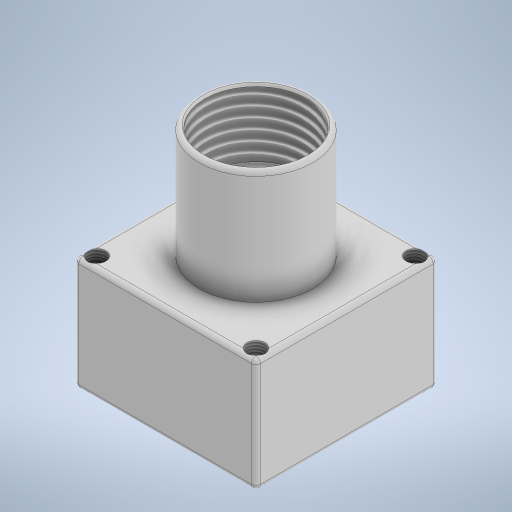
# Autodesk Inventor part: PRACTICA #1 CONOCIENDO INVENTOR CARLOS LUCERO NO. 1184321
Saved by Autodesk Inventor 2024 (Build 280153000, 153)
## iProperties
Created: 2024-01-26
Part Number: PRACTICA #1 CONOCIENDO INVENTOR CARLOS LUCERO NO. 1184321
Material: Genérico
Document SubType Name: Modeling
Designer: Andres
Density: 1 g/cm^3
Appearance: Valor por defecto
Author: Andres
Autodesk Inventor part; units mm, degrees
ref_plane "YZ Plane" through (0, 0, 0) normal (1, 0, 0) x (0, 1, 0)
ref_plane "XZ Plane" through (0, 0, 0) normal (0, 1, 0) x (-1, 0, 0)
ref_plane "XY Plane" through (0, 0, 0) normal (0, 0, 1) x (1, 0, 0)
sketch "Boceto1" plane through (0, 0, 0) normal (0, 1, 0) x (-1, 0, 0)
  line L0 (40, 40) -> (-40, 40)
  line L1 (-40, 40) -> (-40, -40)
  line L2 (-40, -40) -> (40, -40)
  line L3 (40, -40) -> (40, 40)
  line L4 (40, 40) -> (-40, -40) construction
  line L5 (-40, 40) -> (40, -40) construction
  point P0 (0, 0)
  dimension "d0" = 80
  dimension "d1" = 80
  constraints: 12 end point, 2 midpoint, 2 parallel, 1 horizontal, 1 perpendicular
  measures "d0" distance of L0.start L0.end
  measures "d1" distance of L1.end L0.end
extrude "Extrusión1" add sketch "Boceto1" along normal blind 50
sketch "Boceto2" plane through (0, 50, 0) normal (0, 1, 0) x (1, 0, 0)
  circle A0 centre (0, 0) radius 25
  circle A1 centre (0, 0) radius 22.5
  dimension "d4" = 50
  dimension "d5" = 45
  constraints: 2 centre point, 2 coincident
  measures "d4" diameter of A0
  measures "d5" diameter of A1
extrude "Extrusión2" add sketch "Boceto2" along normal blind 50 contours A0 | A1
sketch "Boceto3" plane through (0, 100, 0) normal (0, 1, 0) x (1, 0, 0)
  circle A0 centre (0, 0) radius 22.5
  dimension "d8" = 45
  constraints: 1 centre point, 1 coincident
  measures "d8" diameter of A0
extrude "Extrusión3" cut sketch "Boceto3" against normal blind 30
sketch "Boceto4" plane through (0, 0, 0) normal (0, -1, 0) x (1, 0, 0)
  line L0 (35, 35) -> (-35, 35)
  line L1 (-35, 35) -> (-35, -35)
  line L2 (-35, -35) -> (35, -35)
  line L3 (35, -35) -> (35, 35)
  line L4 (35, 35) -> (-35, -35) construction
  line L5 (-35, 35) -> (35, -35) construction
  circle A0 centre (35, 35) radius 4
  circle A1 centre (35, -35) radius 4
  circle A2 centre (-35, -35) radius 4
  circle A3 centre (-35, 35) radius 4
  point P0 (0, 0)
  dimension "d11" = 70
  dimension "d12" = 70
  dimension "d13" = 8
  dimension "d14" = 8
  dimension "d15" = 8
  dimension "d16" = 8
  constraints: 12 end point, 4 centre point, 4 coincident, 2 midpoint, 2 parallel, 1 horizontal, 1 perpendicular
  measures "d11" distance of L0.start L0.end
  measures "d12" distance of L1.end L0.end
  measures "d13" diameter of A0
  measures "d14" diameter of A1
  measures "d15" diameter of A2
  measures "d16" diameter of A3
extrude "Extrusión4" cut sketch "Boceto4" against normal blind 50 contours A0 L3 L0 | L0 L3 A0
sketch "Boceto5" plane through (0, 0, 0) normal (0, -1, 0) x (1, 0, 0)
  line L0 (-35, 35) -> (-31, 35)
  line L1 (35, -31) -> (35, -35)
  line L2 (35, 35) -> (-35, -35) construction
  circle A0 centre (-35, 35) radius 4
  circle A1 centre (-35, -35) radius 4
  circle A2 centre (35, -35) radius 4
  line L3 (35, -35) -> (31, -35)
  line L4 (-31, -35) -> (-35, -35)
  line L5 (-35, -35) -> (-35, -31)
  line L6 (-35, 31) -> (-35, 35)
  point P0 (0, 0)
  dimension "d19" = 70
  dimension "d20" = 70
  dimension "d22" = 8
  dimension "d23" = 8
  constraints: 14 end point, 6 point on circle, 4 parallel, 3 centre point, 3 coincident, 1 horizontal, 1 midpoint, 1 perpendicular
  measures "d19" distance of L0.start L2.start
  measures "d20" distance of L2.start L1.end
  measures "d22" diameter of A1
  measures "d23" diameter of A2
extrude "Extrusión5" cut sketch "Boceto5" against normal blind 50 contours L6 A0 L0 | L0 A0 L6
sketch "Boceto6" plane through (0, 0, 0) normal (0, -1, 0) x (1, 0, 0)
  line L0 (-35, 35) -> (35, 35)
  line L1 (35, 35) -> (35, -35)
  line L2 (35, -35) -> (-35, -35)
  line L3 (-35, -35) -> (-35, 35)
  line L4 (-35, 35) -> (35, -35) construction
  line L5 (35, 35) -> (-35, -35) construction
  circle A0 centre (35, -35) radius 4
  circle A1 centre (-35, -35) radius 4
  point P0 (0, 0)
  dimension "d26" = 70
  dimension "d27" = 70
  dimension "d28" = 8
  dimension "d29" = 8
  constraints: 12 end point, 2 centre point, 2 coincident, 2 midpoint, 2 parallel, 1 horizontal, 1 perpendicular
  measures "d26" distance of L0.start L0.end
  measures "d27" distance of L0.end L1.end
  measures "d28" diameter of A0
  measures "d29" diameter of A1
extrude "Extrusión6" cut sketch "Boceto6" against normal blind 50 contours A1 L2 L3 | L3 L2 A1 | A0 L2 L1 | L1 L2 A0
thread "Rosca1" size "M45x4.5" class "6H" standard "ANSI Metric M Profile" full length
thread "Rosca2" size "M8x1.25" class "6H" standard "ANSI Metric M Profile" full length
thread "Rosca3" size "M8x1.25" class "6H" standard "ANSI Metric M Profile" full length
thread "Rosca4" size "M8x1.25" class "6H" standard "ANSI Metric M Profile" full length
fillet "Empalme1" radius 2 14 edges at (0, 50, -40) (-40, 25, -40) (-40, 50, 0) (-40, 25, 40) (40, 25, -40) (40, 50, 0) (40, 25, 40) (0, 50, 40) (0, 0, 40) (40, 0, 0) (0, 0, -40) (-40, 0, 0) (-25, 100, 0) (-22.5, 100, 0)
